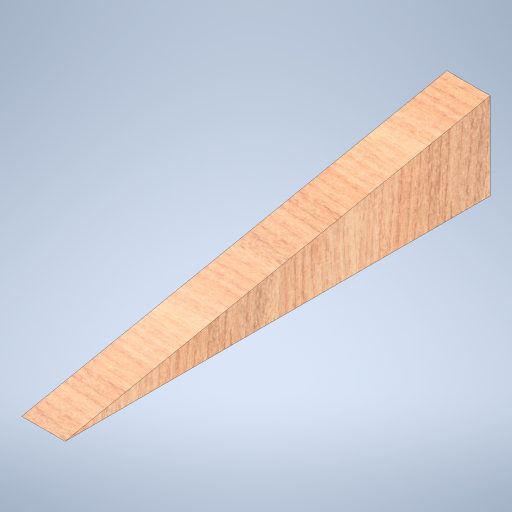
# Autodesk Inventor part: boardBaseWedge
Saved by Autodesk Inventor 2024.2 (Build 282272000, 272)
## iProperties
Created: 2024-06-09
Part Number: boardBaseWedge
Material: Wood (Birch)
Document SubType Name: Modeling
Designer: user
Density: 0.55 g/cm^3
Appearance: Birch - Natural Polished
Author: user
Autodesk Inventor part; units mm, degrees
ref_plane "YZ Plane" through (0, 0, 0) normal (1, 0, 0) x (0, 1, 0)
ref_plane "XZ Plane" through (0, 0, 0) normal (0, 1, 0) x (-1, 0, 0)
ref_plane "XY Plane" through (0, 0, 0) normal (0, 0, 1) x (1, 0, 0)
sketch "Sketch2" plane through (0, 0, 0) normal (1, 0, 0) x (0, 1, 0)
  line L0 (0, 0) -> (0, 489.8979)
  line L1 (0, 489.8979) -> (100, 0)
  line L2 (100, 0) -> (0, 0)
  dimension "d0" = 500
  dimension "d2" = 100
  constraints: 6 end point, 1 perpendicular, 1 vertical
  measures "d0" distance of L0.end L1.end
  measures "d2" distance of L1.end L0.start
extrude "Extrusion1" add sketch "Sketch2" along normal blind 50
body "Solid1"
